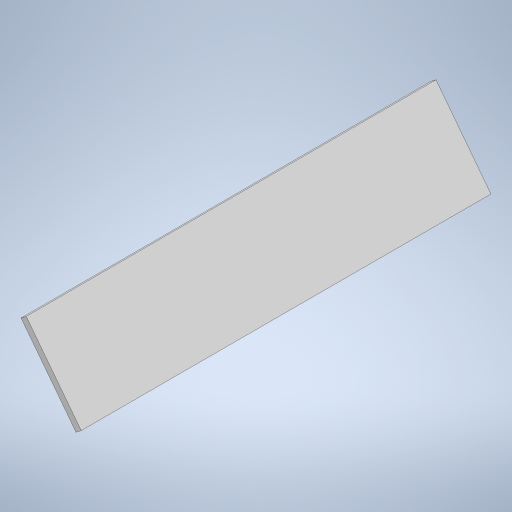
# Autodesk Inventor part: Part8
Saved by Autodesk Inventor 2023 (Build 270158000, 158)
## iProperties
Created: 2024-03-19
Part Number: Part8
Material: Generic
Document SubType Name: Modeling
Designer: noname
Density: 1 g/cm^3
Appearance: Default
Author: noname
Autodesk Inventor part; units mm, degrees
ref_plane "YZ Plane" through (0, 0, 0) normal (1, 0, 0) x (0, 1, 0)
ref_plane "XZ Plane" through (0, 0, 0) normal (0, 1, 0) x (-1, 0, 0)
sketch "Sketch2" plane through (0, 0, 0) normal (0, 0, 1) x (1, 0, 0)
  line L0 (12.1829, -15.8377) -> (-1.2308, 1.6)
  line L1 (-1.2308, 1.6) -> (-2.499, 0.6245)
  line L2 (-2.499, 0.6245) -> (10.9147, -16.8133)
  line L3 (10.9147, -16.8133) -> (12.1829, -15.8377)
  line L4 (12, -15.6) -> (100, -15.6) projected
  line L5 (100, -15.6) -> (100, -14) projected
  line L6 (12, -14) -> (100, -14) projected
  line L7 (12, -15.6) -> (12, -14) projected
  line L8 (0, 0) -> (100, 0) projected
  line L9 (100, 0) -> (100, 1.6) projected
  line L10 (0, 1.6) -> (100, 1.6) projected
  line L11 (0, 0) -> (0, 1.6) projected
  dimension "d0" = 1.6
  dimension "d1" = 22
  constraints: 8 end point, 2 parallel, 2 point on line, 1 horizontal alignment, 1 perpendicular
  measures "d0" distance between parallel lines of L2 L0
  measures "d1" distance between parallel lines of L1 L3
ref_plane "Work Plane1" through (15, -19.5, -83) normal (0, 0, -1) x (0, 1, 0)
extrude "Extrusion1" add sketch "Sketch2" against normal blind 100 contours L3 L2 L1 L0
body "Solid1"
